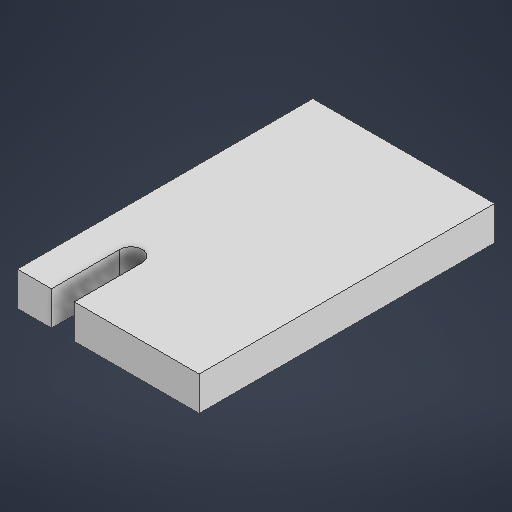
# Autodesk Inventor part: Part4
Saved by Autodesk Inventor 2026 (Build 300175050, 175E)
## iProperties
Created: 2026-04-16
Part Number: Part4
Material: Generic
Document SubType Name: Modeling
Designer: Administrator
Density: 1 g/cm^3
Appearance: Default
Author: Administrator
Autodesk Inventor part; units mm, degrees
ref_plane "YZ Plane" through (0, 0, 0) normal (1, 0, 0) x (0, 1, 0)
ref_plane "XZ Plane" through (0, 0, 0) normal (0, 1, 0) x (-1, 0, 0)
ref_plane "XY Plane" through (0, 0, 0) normal (0, 0, 1) x (1, 0, 0)
sketch "Sketch1" plane through (0, 0, 0) normal (0, 1, 0) x (-1, 0, 0)
  line L0 (0, 0) -> (0, -130)
  line L1 (0, -130) -> (80, -130)
  line L2 (80, -130) -> (80, 0)
  line L3 (80, 0) -> (0, 0)
  dimension "d0" = 130
  dimension "d1" = 80
  constraints: 8 end point, 3 perpendicular, 1 vertical
  measures "d0" distance of L0.start L0.end
  measures "d1" distance of L0.end L1.end
extrude "Extrusion1" add sketch "Sketch1" along normal mid plane 15
sketch "Sketch2" plane through (0, 7.5, 0) normal (0, 1, 0) x (1, 0, 0)
  line L0 (-60, -12.1758) -> (-60, 30) construction
  line L1 (-55, -12.1758) -> (-55, 30)
  line L2 (-65, 30) -> (-65, -12.1758)
  arc A0 (-65, -12.1758) -> (-55, -12.1758) centre (-60, -12.1758) ccw
  arc A1 (-55, 30) -> (-65, 30) centre (-60, 30) ccw
  line L3 (-80, 130) -> (-80, 0) projected
  line L4 (-80, 0) -> (0, 0) projected
  point P0 (-60, 8.9121)
  point P1 (-65, 0)
  point P2 (-55, 0)
  dimension "d4" = 10
  dimension "d5" = 20
  dimension "d6" = 30
  constraints: 8 end point, 4 point on circle, 4 tangent, 2 centre point, 1 midpoint, 1 parallel, 1 vertical
  measures "d4" diameter of A1
  measures "d5" distance between parallel lines of L3 L0
  measures "d6" distance from line of L0.end L4
extrude "Extrusion2" cut sketch "Sketch2" along normal through all both and the other way through all contours L4 L2 A1 L1
body "Solid1"
